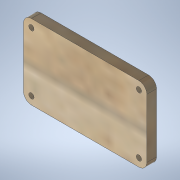
# Autodesk Inventor part: ロボット回転t5.5_2
Saved by Autodesk Inventor 2020.3 (Build 243373000, 373)
## iProperties
Created: 2020-07-07
Part Number: ロボット回転t5.5_2
Material: 木材 (カエデ材)
Document SubType Name: Modeling
Designer: totot
Density: 0.67 g/cm^3
Appearance: ナチュラル カエデ材 - 光沢 濃い着色
Author: totot
Autodesk Inventor part; units mm, degrees
ref_plane "YZ Plane" through (0, 0, 0) normal (1, 0, 0) x (0, 1, 0)
ref_plane "XZ Plane" through (0, 0, 0) normal (0, 1, 0) x (-1, 0, 0)
ref_plane "XY Plane" through (0, 0, 0) normal (0, 0, 1) x (1, 0, 0)
sketch "スケッチ1" plane through (0, 0, 0) normal (0, 0, 1) x (1, 0, 0)
  line L0 (0, 0) -> (70, 0)
  line L1 (70, 0) -> (70, -42.5)
  line L2 (70, -42.5) -> (0, -42.5)
  line L3 (0, -42.5) -> (0, 0)
  dimension "d0" = 70
  dimension "d1" = 42.5
  constraints: 8 end point, 2 parallel, 1 horizontal, 1 perpendicular
  measures "d0" distance of L1.end L2.end
  measures "d1" distance of L0.end L1.end
extrude "押し出し1" add sketch "スケッチ1" along normal blind 5.5
sketch "スケッチ2" plane through (0, 0, 5.5) normal (0, 0, 1) x (1, 0, 0)
  line L0 (4.5, -38) -> (65.5, -38)
  line L1 (65.5, -38) -> (65.5, -4.5)
  line L2 (65.5, -4.5) -> (4.5, -4.5)
  line L3 (4.5, -4.5) -> (4.5, -38)
  line L4 (0, 0) -> (0, -42.5) projected
  line L5 (0, -42.5) -> (70, -42.5) projected
  dimension "d4" = 61
  dimension "d5" = 33.5
  dimension "d6" = 4.5
  dimension "d7" = 4.5
  constraints: 8 end point, 4 coincident, 2 parallel, 1 horizontal, 1 perpendicular
  measures "d4" distance of L2.end L1.end
  measures "d5" distance of L1.end L0.end
  measures "d6" distance between parallel lines of L3 L4
  measures "d7" distance between parallel lines of L0 L5
hole "穴1" at (4.5, -38, 5.5) at (4.5, -4.5, 5.5) at (65.5, -4.5, 5.5) at (65.5, -38, 5.5) direction (0, 0, -1) diameter 3 end through all
fillet "フィレット1" radius 4.5 4 edges at (0, 0, 2.75) (70, 0, 2.75) (70, -42.5, 2.75) (0, -42.5, 2.75)
sketch "スケッチ3" plane through (0, 0, 5.5) normal (0, 0, 1) x (1, 0, 0)
  line L0 (65.5, 0) -> (4.5, 0) projected
  line L1 (70, -38) -> (70, -4.5) projected
  point P0 (0, 0)
  point P1 (46, -26)
  dimension "d16" = 26
  dimension "d17" = 24
  measures "d16" distance from line of point (46, -26) L0
  measures "d17" distance from line of point (46, -26) L1
hole "穴2" at (46, -26, 5.5) direction (0, 0, -1) diameter 6 end through all
